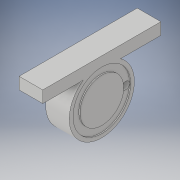
# Autodesk Inventor part: Camera Mount
Saved by Autodesk Inventor 2019 (Build 230136000, 136)
## iProperties
Created: 2019-01-11
Part Number: Camera Mount
Material: Generic
Document SubType Name: Modeling
Designer: pepin
Density: 1 g/cm^3
Appearance: Default
Author: pepin
Autodesk Inventor part; units mm, degrees
ref_plane "YZ Plane" through (0, 0, 0) normal (1, 0, 0) x (0, 1, 0)
ref_plane "XZ Plane" through (0, 0, 0) normal (0, 1, 0) x (-1, 0, 0)
ref_plane "XY Plane" through (0, 0, 0) normal (0, 0, 1) x (1, 0, 0)
sketch "Sketch1" plane through (0, 0, 0) normal (0, 0, 1) x (1, 0, 0)
  line L0 (-12.7, -6.35) -> (12.7, -6.35)
  line L1 (12.7, -6.35) -> (12.7, 6.35)
  line L2 (12.7, 6.35) -> (-12.7, 6.35)
  line L3 (-12.7, 6.35) -> (-12.7, -6.35)
  line L4 (-12.7, -6.35) -> (12.7, 6.35) construction
  line L5 (12.7, -6.35) -> (-12.7, 6.35) construction
  point P0 (0, 0)
  dimension "d0" = 25.4
  dimension "d1" = 12.7
  constraints: 12 end point, 2 midpoint, 2 parallel, 1 horizontal, 1 perpendicular
  measures "d0" distance of L1.end L2.end
  measures "d1" distance of L2.end L0.start
extrude "Extrusion1" add sketch "Sketch1" along normal mid plane 127
sketch "Sketch2" plane through (12.7, -6.35, 63.5) normal (1, 0, 0) x (0, 0, -1)
  line L0 (0, 0) -> (0, 12.7) construction
  line L1 (0, 6.35) -> (127, 6.35) construction
  line L2 (127, 12.7) -> (127, 0) construction
  line L3 (63.5, 6.35) -> (63.5, -28.65) construction
  circle A0 centre (63.5, -28.65) radius 35
  dimension "d4" = 35
  dimension "d5" = 70
  constraints: 4 end point, 2 midpoint, 1 centre point, 1 coincident, 1 vertical
  measures "d4" distance from line of L3.end L1
  measures "d5" diameter of A0
extrude "Extrusion2" add sketch "Sketch2" against normal blind 25.4
sketch "Sketch3" plane through (12.7, -6.35, -63.5) normal (1, 0, 0) x (0, 0, -1)
  circle A0 centre (-63.5, -28.65) radius 0.1553
  line L0 (-63.5, 6.35) -> (-63.5, -28.65) construction
  circle A1 centre (-63.5, -28.65) radius 23.5
  circle A2 centre (-63.5, -28.65) radius 31
  dimension "d8" = 35
  dimension "d9" = 62
  dimension "d10" = 47
  constraints: 3 centre point, 2 coincident, 2 end point, 1 vertical
  measures "d8" distance of L0.start L0.end
  measures "d9" diameter of A2
  measures "d10" diameter of A1
extrude "Extrusion3" cut sketch "Sketch3" against normal blind 1.25 contours A2
sketch "Sketch4" plane through (12.7, -35, 0) normal (1, 0, 0) x (0, 0, -1)
  circle A0 centre (27.0286, -0.3946) radius 4
  point P0 (0, 35)
  dimension "d16" = 8
  constraints: 1 centre point
  measures "d16" diameter of A0
extrude "Extrusion5" cut sketch "Sketch4" against normal blind 25.4
body "Solid1"
